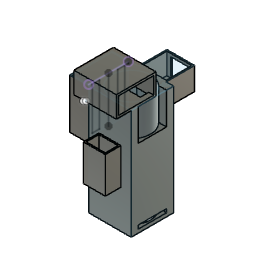
SquareBaseAirHorn (Autodesk Fusion 360 design; units mm, degrees)
Autodesk Fusion 360 part; units mm, degrees
sketch "Sketch1" plane through (0, 0, 0) normal (0, 0, 1) x (1, 0, 0)
  line L0 (0, 0) -> (60, 0)
  line L1 (60, 0) -> (60, -60)
  line L2 (60, -60) -> (0, -60)
  line L3 (0, -60) -> (0, 0)
  dimension "d1" = 60
  dimension "d2" = 60
  constraint horizontal L0
  constraint vertical L1
  constraint horizontal L2
  constraint vertical L3
  constraint coincident L0.start L3.end
  measures "d1" distance of L0.start L0.end
  measures "d2" distance of L0.end L1.end
extrude "Extrude1" add sketch "Sketch1" along normal blind 155
sketch "Sketch2" plane through (0, 0, 0) normal (0, 0, 1) x (1, 0, 0)
  line L0 (0, 0) -> (30, 0)
  line L1 (30, 0) -> (30, -30)
  circle A0 centre (30, -30) radius 27.5
  dimension "d5" = 30
  dimension "d6" = 30
  dimension "d7" = 55
  constraint coincident L0.start origin
  constraint horizontal L0
  constraint perpendicular L0 L1
  constraint coincident L1.end A0.centre
  measures "d5" distance of L0.start L0.end
  measures "d6" distance of L0.end L1.end
  measures "d7" diameter of A0
extrude "Extrude2" cut sketch "Sketch2" along normal through all
sketch "Sketch3" plane through (0, 0, 0) normal (1, 0, 0) x (0, 1, 0)
  line L0 (0, 0) -> (0, 5)
  line L1 (0, 5) -> (-10, 5)
  line L2 (-10, 5) -> (-50, 5)
  line L3 (-50, 5) -> (-50, 10)
  line L4 (-50, 10) -> (-10, 10)
  line L5 (-10, 10) -> (-10, 5)
  dimension "d9" = 10
  dimension "d10" = 5
  dimension "d11" = 40
  dimension "d12" = 5
  constraint coincident L0.start origin
  constraint vertical L0
  constraint perpendicular L0 L1
  constraint horizontal L2
  constraint vertical L3
  constraint horizontal L4
  constraint vertical L5
  measures "d9" distance of L0.end L1.end
  measures "d10" distance of L0.start L0.end
  measures "d11" distance of L1.end L2.end
  measures "d12" distance of L2.end L3.end
extrude "Extrude3" cut sketch "Sketch3" along normal through all
sketch "Sketch4" plane through (0, 0, 0) normal (-1, 0, 0) x (0, -1, 0)
  line L0 (50, 10) -> (50, 5)
  line L1 (50, 5) -> (10, 5)
  line L2 (10, 5) -> (10, 10)
  line L3 (10, 10) -> (50, 10)
  line L4 (0, 0) -> (60, 0)
  line L5 (60, 0) -> (60, 155)
  line L6 (60, 155) -> (0, 155)
  line L7 (0, 155) -> (0, 0)
  line L8 (0, 155) -> (0.01, 155)
  line L9 (0.01, 155) -> (59.91, 155)
  line L10 (59.91, 155) -> (59.91, 85)
  line L11 (59.91, 85) -> (0.01, 85)
  line L12 (0.01, 85) -> (0.01, 155)
  dimension "d14" = 0.01
  dimension "d15" = 59.9
  dimension "d16" = 70
  constraint coincident L6.end L7.start
  constraint horizontal L8
  constraint horizontal L9
  constraint vertical L10
  constraint horizontal L11
  constraint vertical L12
  measures "d14" distance of L6.end L8.end
  measures "d15" distance of L8.end L9.end
  measures "d16" distance of L8.end L11.end
extrude "Extrude4" add sketch "Sketch4" along normal blind 27 contours L6 L9 L10 L11 L12
sketch "Sketch5" plane through (0, 0, 155) normal (0, 0, 1) x (-1, 0, 0)
  circle A0 centre (-30, 30) radius 27.5
  line L0 (0, 60) -> (-60, 60)
  line L1 (-60, 60) -> (-60, 0)
  line L2 (-60, 0) -> (0, 0)
  line L3 (0, 0) -> (0, 0.01)
  line L4 (0, 0.01) -> (27, 0.01)
  line L5 (27, 0.01) -> (27, 59.91)
  line L6 (27, 59.91) -> (0, 59.91)
  line L7 (0, 59.91) -> (0, 60)
  line L8 (27, 0.01) -> (25, 0.01)
  line L9 (25, 0.01) -> (25, 2.01)
  line L10 (25, 2.01) -> (2, 2.01)
  line L11 (2, 2.01) -> (2, 58.01)
  line L12 (2, 58.01) -> (25, 58.01)
  line L13 (25, 58.01) -> (25, 2.01)
  dimension "d19" = 2
  dimension "d20" = 2
  dimension "d21" = 23
  dimension "d22" = 56
  constraint coincident L4.end L5.start
  constraint coincident L4 L8.end
  constraint perpendicular L5 L8
  constraint perpendicular L8 L9
  constraint horizontal L10
  constraint vertical L11
  constraint horizontal L12
  constraint vertical L13
  measures "d19" distance of L8.end L9.end
  measures "d20" distance of L4.end L8.end
  measures "d21" distance of L9.end L10.end
  measures "d22" distance of L9.end L12.end
extrude "Extrude5" cut sketch "Sketch5" against normal blind 65 contours L10 L11 L12 L13
sketch "Sketch6" plane through (0, -60, 0) normal (0, -1, 0) x (1, 0, 0)
  line L0 (0, 0) -> (60, 0)
  line L1 (60, 0) -> (60, 155)
  line L2 (60, 155) -> (0, 155)
  line L3 (0, 155) -> (0, 0)
sketch "Sketch7" plane through (60, 0, 0) normal (1, 0, 0) x (0, 1, 0)
  line L0 (-50, 5) -> (-50, 10)
  line L1 (-50, 10) -> (-10, 10)
  line L2 (-10, 10) -> (-10, 5)
  line L3 (-10, 5) -> (-50, 5)
  line L4 (-60, 0) -> (0, 0)
  line L5 (0, 0) -> (0, 155)
  line L6 (0, 155) -> (-60, 155)
  line L7 (-60, 155) -> (-60, 0)
sketch "Sketch8" plane through (0, -60, 0) normal (0, -1, 0) x (1, 0, 0)
sketch "Sketch9" plane through (0, -60, 0) normal (0, -1, 0) x (1, 0, 0)
sketch "Sketch10" plane through (0, 0, 0) normal (0, 1, 0) x (-1, 0, 0)
  line L0 (-60, 0) -> (0, 0)
  line L1 (0, 0) -> (0, 155)
  line L2 (0, 155) -> (-60, 155)
  line L3 (-60, 155) -> (-60, 0)
  line L4 (0, 155) -> (-10.5, 155)
  line L5 (-10.5, 155) -> (-49.5, 155)
  line L6 (-49.5, 155) -> (-49.5, 123)
  line L7 (-49.5, 123) -> (-10.5, 123)
  line L8 (-10.5, 123) -> (-10.5, 155)
  dimension "d25" = 10.5
  dimension "d26" = 39
  dimension "d27" = 32
  constraint coincident L1.end L2.start
  constraint perpendicular L1 L4
  constraint horizontal L5
  constraint vertical L6
  constraint horizontal L7
  constraint vertical L8
  measures "d25" distance of L1.end L4.end
  measures "d26" distance of L4.end L5.end
  measures "d27" distance of L5.end L6.end
extrude "Extrude6" add sketch "Sketch10" along normal blind 40 contours L2 L5 L6 L7 L8
sketch "Sketch11" plane through (0, 0, 155) normal (0, 0, 1) x (-1, 0, 0)
  line L0 (2, 2.01) -> (2, 58.01)
  line L1 (2, 58.01) -> (25, 58.01)
  line L2 (25, 58.01) -> (25, 2.01)
  line L3 (25, 2.01) -> (2, 2.01)
  circle A0 centre (-30, 30) radius 27.5
  line L4 (0, 60) -> (-60, 60)
  line L5 (-60, 60) -> (-60, 0)
  line L6 (-60, 0) -> (-49.5, 0)
  line L7 (-49.5, 0) -> (-49.5, -40)
  line L8 (-49.5, -40) -> (-10.5, -40)
  line L9 (-10.5, -40) -> (-10.5, 0)
  line L10 (-10.5, 0) -> (0, 0)
  line L11 (0, 0) -> (0, 0.01)
  line L12 (0, 0.01) -> (27, 0.01)
  line L13 (27, 0.01) -> (27, 59.91)
  line L14 (27, 59.91) -> (0, 59.91)
  line L15 (0, 59.91) -> (0, 60)
sketch "Sketch12" plane through (0, 0, 155) normal (0, 0, 1) x (-1, 0, 0)
sketch "Sketch13" plane through (0, 0, 155) normal (0, 0, 1) x (-1, 0, 0)
sketch "Sketch15" plane through (0, 0, 155) normal (0, 0, 1) x (-1, 0, 0)
  line L0 (-49.5, 0) -> (-47.5, 0)
  line L1 (-47.5, 0) -> (-47.5, -2)
  line L2 (-60, 0) -> (-49.5, 0)
  line L3 (-49.5, 0) -> (-49.5, -40)
  line L4 (-47.5, -2) -> (-12.5, -2)
  line L5 (-12.5, -2) -> (-12.5, -38)
  line L6 (-12.5, -38) -> (-47.5, -38)
  line L7 (-47.5, -38) -> (-47.5, -2)
  dimension "d34" = 2
  dimension "d35" = 2
  dimension "d36" = 35
  dimension "d37" = 36
  constraint horizontal L0
  constraint perpendicular L0 L1
  constraint coincident L0.start L2
  constraint coincident L0.start L3
  constraint horizontal L4
  constraint vertical L5
  constraint horizontal L6
  constraint vertical L7
  measures "d34" distance of L0.start L0.end
  measures "d35" distance of L0.end L1.end
  measures "d36" distance of L1.end L4.end
  measures "d37" distance of L4.end L5.end
extrude "Extrude7" cut sketch "Sketch15" against normal blind 30
sketch "Sketch16" plane through (0, 40, 0) normal (0, 1, 0) x (-1, 0, 0)
  line L0 (-10.5, 123) -> (-10.5, 155)
  line L1 (-10.5, 155) -> (-49.5, 155)
  line L2 (-49.5, 155) -> (-49.5, 123)
  line L3 (-49.5, 123) -> (-10.5, 123)
  line L4 (-49.5, 155) -> (-42, 155)
  line L5 (-42, 155) -> (-42, 151)
  line L6 (-42, 151) -> (-18, 151)
  line L7 (-18, 151) -> (-18, 127)
  line L8 (-18, 127) -> (-42, 127)
  line L9 (-42, 127) -> (-42, 151)
  dimension "d40" = 7.5
  dimension "d41" = 4
  dimension "d42" = 24
  dimension "d43" = 24
  constraint coincident L1.end L2.start
  constraint perpendicular L2 L4
  constraint perpendicular L1 L5
  constraint horizontal L6
  constraint vertical L7
  constraint horizontal L8
  constraint vertical L9
  measures "d40" distance of L1.end L4.end
  measures "d41" distance of L4.end L5.end
  measures "d42" distance of L5.end L6.end
  measures "d43" distance of L5.end L8.end
extrude "Extrude8" cut sketch "Sketch16" against normal blind 15 contours L6 L7 L8 L9
sketch "Sketch17" plane through (0, 2, 0) normal (0, 1, 0) x (-1, 0, 0)
  line L0 (-12.5, 155) -> (-47.5, 155)
  line L1 (-47.5, 155) -> (-47.5, 125)
  line L2 (-47.5, 125) -> (-12.5, 125)
  line L3 (-12.5, 125) -> (-12.5, 155)
  line L4 (-47.5, 155) -> (-28, 155)
  line L5 (-28, 155) -> (-28, 139)
  circle A0 centre (-28, 139) radius 5
  dimension "d46" = 19.5
  dimension "d47" = 16
  dimension "d48" = 10
  constraint coincident L0.end L1.start
  constraint perpendicular L1 L4
  constraint perpendicular L0 L5
  constraint coincident L5.end A0.centre
  measures "d46" distance of L0.end L4.end
  measures "d47" distance of L4.end L5.end
  measures "d48" diameter of A0
extrude "Extrude9" cut sketch "Sketch17" against normal blind 12 contours A0
sketch "Sketch18" plane through (0, -60, 0) normal (0, -1, 0) x (1, 0, 0)
sketch "Sketch19" plane through (0, -60, 0) normal (0, -1, 0) x (1, 0, 0)
sketch "Sketch20" plane through (0, -60, 0) normal (0, -1, 0) x (1, 0, 0)
  line L0 (45.5, 105) -> (14.5, 105)
  line L1 (14.5, 105) -> (14.5, 54)
  line L2 (14.5, 54) -> (45.5, 54)
  line L3 (45.5, 54) -> (45.5, 105)
  line L4 (60, 0) -> (60, 155)
  line L5 (45.5, 105) -> (60, 105)
  line L6 (60, 105) -> (60, 155)
  dimension "d52" = 31
  dimension "d53" = 51
  dimension "d96" = 50
  dimension "d97" = 14.5
  constraint horizontal L0
  constraint vertical L1
  constraint horizontal L2
  constraint vertical L3
  constraint coincident L4 L5.end
  constraint perpendicular L4 L5
  constraint coincident L4.end L6.end
  measures "d52" distance of L0.start L0.end
  measures "d53" distance of L0.start L2.end
  measures "d96" distance of L5.end L4.end
  measures "d97" distance of L0.start L5.end
extrude "Extrude10" add sketch "Sketch20" along normal blind 22
sketch "Sketch21" plane through (0, 0, 155) normal (0, 0, 1) x (-1, 0, 0)
  line L0 (-12.5, -2) -> (-12.5, -38)
  line L1 (-12.5, -38) -> (-47.5, -38)
  line L2 (-47.5, -38) -> (-47.5, -2)
  line L3 (-47.5, -2) -> (-12.5, -2)
  line L4 (2, 2.01) -> (2, 58.01)
  line L5 (2, 58.01) -> (25, 58.01)
  line L6 (25, 58.01) -> (25, 2.01)
  line L7 (25, 2.01) -> (2, 2.01)
  circle A0 centre (-30, 30) radius 27.5
  line L8 (0, 60) -> (-60, 60)
  line L9 (-60, 60) -> (-60, 0)
  line L10 (-60, 0) -> (-49.5, 0)
  line L11 (-49.5, 0) -> (-49.5, -40)
  line L12 (-49.5, -40) -> (-10.5, -40)
  line L13 (-10.5, -40) -> (-10.5, 0)
  line L14 (-10.5, 0) -> (0, 0)
  line L15 (0, 0) -> (0, 0.01)
  line L16 (0, 0.01) -> (27, 0.01)
  line L17 (27, 0.01) -> (27, 59.91)
  line L18 (27, 59.91) -> (0, 59.91)
  line L19 (0, 59.91) -> (0, 60)
  line L20 (-14.5, 82) -> (-14.5, 80)
  line L21 (-14.5, 80) -> (-16.5, 80)
  dimension "d56" = 2
  dimension "d57" = 2
  constraint perpendicular L20 L21
  measures "d56" distance of L20.start L20.end
  measures "d57" distance of L20.end L21.end
sketch "Sketch22" plane through (0, 0, 155) normal (0, 0, 1) x (-1, 0, 0)
  line L0 (-16.5, 80) -> (-43.5, 80)
  line L1 (-43.5, 80) -> (-43.5, 62)
  line L2 (-43.5, 62) -> (-16.5, 62)
  line L3 (-16.5, 62) -> (-16.5, 80)
  dimension "d58" = 27
  dimension "d59" = 18
  constraint horizontal L0
  constraint vertical L1
  constraint horizontal L2
  constraint vertical L3
  measures "d58" distance of L0.start L0.end
  measures "d59" distance of L0.start L2.end
extrude "Extrude11" cut sketch "Sketch22" against normal blind 99
sketch "Sketch23" plane through (0, 0, 155) normal (0, 0, 1) x (-1, 0, 0)
sketch "Sketch24" plane through (0, 0, 155) normal (0, 0, 1) x (1, 0, 0)
sketch "Sketch26" plane through (-2, 0, 0) normal (-1, 0, 0) x (0, -1, 0)
  line L0 (58.01, 155) -> (2.01, 155)
  line L1 (2.01, 155) -> (2.01, 90)
  line L2 (2.01, 90) -> (58.01, 90)
  line L3 (58.01, 90) -> (58.01, 155)
  line L4 (2.01, 155) -> (2.01, 153)
  line L5 (2.01, 153) -> (7.01, 153)
  line L6 (7.01, 153) -> (17.01, 153)
  line L7 (17.01, 153) -> (17.01, 93)
  line L8 (17.01, 93) -> (7.01, 93)
  line L9 (7.01, 93) -> (7.01, 153)
  line L10 (30.01, 155) -> (30.01, 90)
  line L11 (2.01, 155) -> (58.01, 155)
  line L12 (43.01, 153) -> (43.01, 93)
  line L13 (53.01, 153) -> (43.01, 153)
  line L14 (53.01, 93) -> (53.01, 153)
  line L15 (43.01, 93) -> (53.01, 93)
  dimension "d66" = 2
  dimension "d67" = 5
  dimension "d68" = 10
  dimension "d69" = 60
  constraint coincident L0.end L1.start
  constraint perpendicular L0 L4
  constraint perpendicular L4 L5
  constraint horizontal L6
  constraint vertical L7
  constraint horizontal L8
  constraint vertical L9
  constraint coincident L0 L10.start
  constraint coincident L2 L10.end
  constraint perpendicular L2 L10
  constraint midpoint L10.start L11
  constraint symmetric L5.end L10 L13.start
  constraint symmetric L6.end L10 L12.start
  constraint symmetric L7.end L10 L12.end
  constraint symmetric L8.end L10 L14.start
  measures "d66" distance of L0.end L4.end
  measures "d67" distance of L4.end L5.end
  measures "d68" distance of L5.end L6.end
  measures "d69" distance of L5.end L8.end
extrude "Extrude14" cut sketch "Sketch26" against normal blind 25 contours L12 L13 L14 L15
extrude "Extrude13" cut sketch "Sketch26" against normal blind 25 contours L6 L7 L8 L9
sketch "Sketch27" plane through (60, 0, 0) normal (1, 0, 0) x (0, 1, 0)
  line L0 (-60, 155) -> (-50, 155)
  line L1 (-50, 155) -> (-10, 155)
  line L2 (-10, 155) -> (-10, 110)
  line L3 (-10, 110) -> (-50, 110)
  line L4 (-50, 110) -> (-50, 155)
  dimension "d74" = 10
  dimension "d75" = 40
  dimension "d76" = 45
  constraint horizontal L0
  constraint horizontal L1
  constraint vertical L2
  constraint horizontal L3
  constraint vertical L4
  measures "d74" distance of L0.start L0.end
  measures "d75" distance of L0.end L1.end
  measures "d76" distance of L0.end L3.end
extrude "Extrude15" cut sketch "Sketch27" against normal blind 20
sketch "Sketch28" plane through (0, 0, 155) normal (0, 0, 1) x (-1, 0, 0)
  line L0 (-60, 30) -> (0, 30) construction
  line L1 (-60, 60) -> (-60, 0)
  line L2 (0, 30) -> (0, 25)
  line L3 (0, 25) -> (-60, 25)
  line L4 (-60, 25) -> (-60, 81)
  line L5 (-60, 81) -> (0, 81)
  line L6 (0, 81) -> (0, 25)
  dimension "d79" = 5
  dimension "d80" = 60
  dimension "d81" = 56
  constraint horizontal L0
  constraint midpoint L0.start L1
  constraint perpendicular L0 L2
  constraint horizontal L3
  constraint vertical L4
  constraint horizontal L5
  constraint vertical L6
  measures "d79" distance of L0.end L2.end
  measures "d80" distance of L2.end L3.end
  measures "d81" distance of L2.end L5.end
extrude "Extrude16" add sketch "Sketch28" along normal blind 30
sketch "Sketch29" plane through (0, 0, 155) normal (0, 0, 1) x (-1, 0, 0)
sketch "Sketch30" plane through (0, 0, 0) normal (-1, 0, 0) x (0, -1, 0)
  line L0 (59.91, 155) -> (59.91, 85)
  line L1 (59.91, 85) -> (0.01, 85)
  line L2 (0.01, 85) -> (0.01, 155)
  line L3 (0.01, 155) -> (0, 155)
  line L4 (0, 155) -> (0, 0)
  line L5 (0, 0) -> (60, 0)
  line L6 (60, 0) -> (60, 155)
  line L7 (60, 155) -> (81, 155)
  line L8 (81, 155) -> (81, 185)
  line L9 (81, 185) -> (25, 185)
  line L10 (25, 185) -> (25, 155)
  line L11 (25, 155) -> (59.91, 155)
  line L12 (50, 10) -> (50, 5)
  line L13 (50, 5) -> (10, 5)
  line L14 (10, 5) -> (10, 10)
  line L15 (10, 10) -> (50, 10)
  line L16 (25, 185) -> (28, 185)
  line L17 (28, 185) -> (28, 182)
  line L18 (28, 182) -> (78, 182)
  line L19 (78, 182) -> (78, 158)
  line L20 (78, 158) -> (28, 158)
  line L21 (28, 158) -> (28, 182)
  dimension "d84" = 3
  dimension "d85" = 3
  dimension "d86" = 50
  dimension "d87" = 24
  constraint coincident L9.end L10.start
  constraint coincident L9 L16.end
  constraint perpendicular L9 L17
  constraint horizontal L18
  constraint vertical L19
  constraint horizontal L20
  constraint vertical L21
  measures "d84" distance of L9.end L16.end
  measures "d85" distance of L16.end L17.end
  measures "d86" distance of L17.end L18.end
  measures "d87" distance of L17.end L20.end
extrude "Extrude17" cut sketch "Sketch30" against normal through all contours L18 L19 L20 L21
sketch "Sketch31" plane through (60, 0, 0) normal (1, 0, 0) x (0, 1, 0)
sketch "Sketch32" plane through (0, 0, 185) normal (0, 0, 1) x (-1, 0, 0)
  line L0 (0, 81) -> (-60, 81)
  line L1 (-60, 81) -> (-60, 25)
  line L2 (-60, 25) -> (0, 25)
  line L3 (0, 25) -> (0, 81)
  line L4 (0, 25) -> (-60, 25)
  line L5 (-60, 25) -> (-60, 48)
  line L6 (-60, 48) -> (0, 48)
  line L7 (0, 48) -> (0, 25)
  dimension "d89" = 60
  dimension "d90" = 23
  constraint horizontal L4
  constraint vertical L5
  constraint horizontal L6
  constraint vertical L7
  constraint coincident L2.end L3.start
  measures "d89" distance of L2.end L1.end
  measures "d90" distance of L2.end L6.end
sketch "Sketch33" plane through (0, 0, 158) normal (0, 0, 1) x (-1, 0, 0)
  line L0 (-60, 78) -> (-60, 28)
  line L1 (-60, 28) -> (0, 28)
  line L2 (0, 28) -> (0, 78)
  line L3 (0, 78) -> (-60, 78)
  line L4 (0, 28) -> (-5, 28)
  line L5 (-5, 28) -> (-53, 28)
  line L6 (-53, 28) -> (-53, 40)
  line L7 (-53, 40) -> (-5, 40)
  line L8 (-5, 40) -> (-5, 28)
  dimension "d93" = 48
  dimension "d94" = 12
  constraint coincident L1.end L2.start
  constraint coincident L1 L4.end
  constraint perpendicular L2 L4
  constraint horizontal L5
  constraint vertical L6
  constraint horizontal L7
  constraint vertical L8
  measures "d93" distance of L4.end L5.end
  measures "d94" distance of L4.end L7.end
extrude "Extrude19" cut sketch "Sketch33" against normal through all contours L1 L5 L6 L7 L8
equation "d60 = -49.00 mm - 50 mm"
